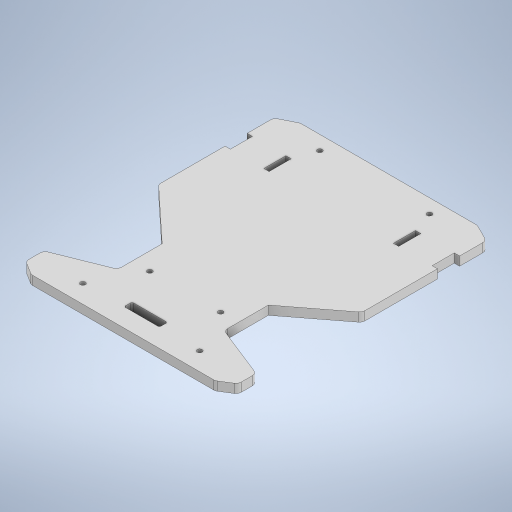
# Autodesk Inventor part: KhungDuoi
Saved by Autodesk Inventor 2023 (Build 270158000, 158)
## iProperties
Created: 2023-03-06
Part Number: KhungDuoi
Material: Generic
Document SubType Name: Modeling
Designer: Admins
Density: 1 g/cm^3
Appearance: Default
Author: Admins
Autodesk Inventor part; units mm, degrees
ref_plane "YZ Plane" through (0, 0, 0) normal (1, 0, 0) x (0, 1, 0)
ref_plane "XZ Plane" through (0, 0, 0) normal (0, 1, 0) x (-1, 0, 0)
ref_plane "XY Plane" through (0, 0, 0) normal (0, 0, 1) x (1, 0, 0)
sketch "Sketch1" plane through (0, 0, 0) normal (0, 1, 0) x (-1, 0, 0)
  line L0 (-60, 75) -> (60, 75)
  line L1 (60, -75) -> (-60, -75)
  line L2 (-60, 75) -> (60, -75) construction
  line L3 (60, 75) -> (-60, -75) construction
  line L4 (-60, -75) -> (-60, -55)
  line L5 (-60, -55) -> (-57, -55)
  line L6 (-60, -55) -> (-57, -55)
  line L7 (-57, -55) -> (-57, -42.5)
  line L8 (-57, -42.5) -> (-60, -42.5)
  line L9 (-60, -42.5) -> (-60, -55)
  line L10 (-57, -42.5) -> (-38.1, -42.5)
  line L11 (-38.1, -42.5) -> (-35.1, -42.5)
  line L12 (-35.1, -42.5) -> (-35.1, -55)
  line L13 (-35.1, -55) -> (-38.1, -55)
  line L14 (-38.1, -55) -> (-38.1, -42.5)
  line L15 (0, 75) -> (0, 64.8)
  line L16 (0, 64.8) -> (-33, 64.8)
  line L17 (-33, 64.8) -> (33, 64.8)
  circle A0 centre (-33, 64.8) radius 1.4
  circle A1 centre (33, 64.8) radius 1.4
  line L18 (0, 75) -> (0, 40)
  line L19 (0, 40) -> (-20, 40)
  line L20 (-20, 40) -> (20, 40)
  circle A2 centre (20, 40) radius 1.4
  circle A3 centre (-20, 40) radius 1.4
  line L21 (-60, -75) -> (-60, -5)
  line L22 (-4, -5) -> (4, -5)
  line L23 (-60, 75) -> (-60, 60)
  line L24 (-60, 60) -> (60, 60)
  line L25 (-20, 40) -> (-21.4, 40)
  line L26 (20, 40) -> (21.4, 40)
  line L27 (-30, 40) -> (-30, 10)
  line L28 (-30, 10) -> (-60, 0)
  line L29 (30, 40) -> (30, 10)
  line L30 (30, 10) -> (60, -5)
  line L31 (-30, 40) -> (-30, 48)
  line L32 (-30, 48) -> (-60, 60)
  line L33 (30, 40) -> (30, 48)
  line L34 (30, 48) -> (60, 60)
  line L35 (0, 75) -> (0, -75)
  line L36 (0, -75) -> (-60, -75)
  line L37 (0, 75) -> (-60, 75)
  line L38 (60, -70) -> (60, -55)
  line L39 (60, -55) -> (57, -55)
  line L40 (57, -55) -> (57, -42.5)
  line L41 (57, -42.5) -> (60, -42.5)
  line L42 (60, -42.5) -> (60, -55)
  line L43 (57, -42.5) -> (38.1, -42.5)
  line L44 (38.1, -42.5) -> (35.1, -42.5)
  line L45 (35.1, -42.5) -> (35.1, -55)
  line L46 (35.1, -55) -> (38.1, -55)
  line L47 (38.1, -55) -> (38.1, -42.5)
  line L48 (60, 75) -> (52, 75)
  line L49 (52, 75) -> (52, 70)
  line L50 (52, 70) -> (60, 70)
  line L51 (60, 70) -> (60, 75)
  line L52 (-60, 75) -> (-52, 75)
  line L53 (-52, 75) -> (-52, 70)
  line L54 (-52, 70) -> (-60, 70)
  line L55 (-60, 70) -> (-60, 75)
  line L56 (60, 70) -> (52, 75)
  line L57 (-52, 75) -> (-60, 70)
  line L58 (60, 75) -> (60, 60)
  line L59 (60, -5) -> (60, -70)
  line L60 (-60, -75) -> (-60, 0)
  line L61 (-60, 60) -> (-60, 75)
  line L62 (57, -75) -> (50, -75)
  line L63 (50, -75) -> (50, -70)
  line L64 (50, -70) -> (60, -70)
  line L65 (60, -70) -> (60, -75)
  line L66 (-60, -75) -> (-50, -75)
  line L67 (-50, -75) -> (-50, -70)
  line L68 (-50, -70) -> (-60, -70)
  line L69 (-60, -70) -> (-60, -75)
  line L70 (-60, -70) -> (-50, -75)
  line L71 (60, -70) -> (50, -75)
  line L72 (33, 64.8) -> (33, 62.8)
  line L73 (33, 62.8) -> (-33, 62.8)
  line L74 (-33, 62.8) -> (-33, 64.8)
  line L75 (0, 62.8) -> (10, 62.8)
  line L76 (10, 62.8) -> (-10, 62.8)
  line L77 (-10, 61.05) -> (10, 61.05)
  line L78 (10, 61.05) -> (10, 64.55)
  line L79 (10, 64.55) -> (-10, 64.55)
  line L80 (-10, 64.55) -> (-10, 61.05)
  line L81 (-10, 61.05) -> (10, 64.55) construction
  line L82 (10, 61.05) -> (-10, 64.55) construction
  line L83 (10, 61.05) -> (-10, 61.05)
  line L84 (-10, 61.05) -> (-10, 60)
  line L85 (-10, 60) -> (10, 60)
  line L86 (10, 60) -> (10, 61.05)
  line L87 (30, 48) -> (30, 23)
  line L88 (30, 23) -> (60, -5)
  line L89 (-30, 48) -> (-30, 23)
  line L90 (-30, 23) -> (-60, 0)
  line L91 (60, -75) -> (31, -75)
  line L92 (31, -75) -> (31, -67)
  line L93 (31, -67) -> (60, -67)
  line L94 (60, -67) -> (60, -75)
  line L95 (-60, -75) -> (-31, -75)
  line L96 (-31, -75) -> (-31, -67)
  line L97 (-31, -67) -> (-60, -67)
  line L98 (-60, -67) -> (-60, -75)
  circle A4 centre (-31, -67) radius 1.4
  circle A5 centre (31, -67) radius 1.4
  point P0 (0, 0)
  dimension "d16" = 2.8
  dimension "d17" = 2.8
  dimension "d0" = 120
  dimension "d1" = 150
  dimension "d2" = 20
  dimension "d3" = 3
  dimension "d4" = 3
  dimension "d5" = 12.5
  dimension "d6" = 18.9
  dimension "d7" = 3
  dimension "d8" = 10.2
  dimension "d9" = 33
  dimension "d10" = 66
  dimension "d11" = 2.8
  dimension "d12" = 2.8
  dimension "d13" = 35
  dimension "d14" = 20
  dimension "d15" = 40
  dimension "d18" = 70
  dimension "d19" = 15
  dimension "d20" = 10
  dimension "d21" = 10
  dimension "d22" = 30
  dimension "d23" = 30
  dimension "d24" = 8
  dimension "d25" = 8
  dimension "d26" = 20
  dimension "d27" = 3
  dimension "d28" = 12.5
  dimension "d29" = 18.9
  dimension "d30" = 3
  dimension "d31" = 8
  dimension "d32" = 5
  dimension "d33" = 8
  dimension "d34" = 5
  dimension "d35" = 10
  dimension "d36" = 5
  dimension "d37" = 10
  dimension "d38" = 5
  dimension "d42" = 2
  dimension "d43" = 10
  dimension "d44" = 20
  dimension "d45" = 3.5
  dimension "d47" = 25
  dimension "d48" = 25
  dimension "d49" = 29
  dimension "d50" = 8
  dimension "d51" = 29
  dimension "d52" = 8
  dimension "d53" = 2.8
  dimension "d54" = 2.8
  constraints: 198 end point, 30 parallel, 23 perpendicular, 17 point on line, 16 horizontal, 7 midpoint, 6 coincident, 4 centre point, 3 vertical, 2 collinear, 2 horizontal alignment, 4 other
  measures "d0" distance of L1.start L1.end
  measures "d1" distance of L0.end L1.start
  measures "d2" distance of L1.end L4.end
  measures "d3" distance of L4.end L5.end
  measures "d4" distance of L8.end L7.end
  measures "d5" distance of L7.end L6.end
  measures "d6" distance of L7.end L10.end
  measures "d7" distance of L12.end L13.end
  measures "d8" distance of L15.start L15.end
  measures "d9" distance of L15.end L16.end
  measures "d10" distance of L16.end L17.end
  measures "d11" diameter of A0
  measures "d12" diameter of A1
  measures "d13" distance of L15.start L18.end
  measures "d14" distance of L18.end L19.end
  measures "d15" distance of L19.end L20.end
  measures "d18" distance of L1.end L21.end
  measures "d19" distance of L0.start L23.end
  measures "d20" distance of L25.start L27.start
  measures "d21" distance of L26.start L29.start
  measures "d22" distance of L27.start L27.end
  measures "d23" distance of L29.start L29.end
  measures "d24" distance of L27.start L31.end
  measures "d25" distance of L29.start L33.end
  measures "d26" distance of L1.start L38.end
  measures "d27" distance of L40.end L41.end
  measures "d28" distance of L39.end L40.end
  measures "d29" distance of L40.end L43.end
  measures "d30" distance of L46.end L45.end
  measures "d31" distance of L50.end L49.end
  measures "d32" distance of L49.end L48.end
  measures "d33" distance of L53.end L54.end
  measures "d34" distance of L52.end L53.end
  measures "d35" distance of L38.start L63.end
  measures "d36" distance of L62.end L63.end
  measures "d37" distance of L68.end L67.end
  measures "d38" distance of L67.end L66.end
  measures "d42" distance of L72.start L72.end
  measures "d43" distance of L75.start L75.end
  measures "d44" distance of L75.end L76.end
  measures "d45" distance of L78.end L77.end
  measures "d47" distance of L33.end L87.end
  measures "d48" distance of L31.end L89.end
  measures "d49" distance of L92.end L93.end
  measures "d50" distance of L91.end L92.end
  measures "d51" distance of L97.end L96.end
  measures "d52" distance of L96.end L95.end
  measures "d53" diameter of A4
  measures "d54" diameter of A5
extrude "Extrusion1" add sketch "Sketch1" along normal blind 5 contours L0 L15 L16 A0 L74 L73 L80 L84 L24 L23 L54 L53 | L53 L54 L57 | L0 L49 L50 L58 L24 L86 L78 L73 L72 A1 L17 L15 | L24 L18 L35 L1 L96 A4 L97 L4 L5 L7 L8 L21 L60 L28 L27 L31 L32 | L56 L50 L49 | L18 L79 L80 L73 L74 A0 L16 | L17 A1 L72 L73 L78 L79 L18 | L24 L34 L33 L29 L30 L59 L41 L40 L39 L38 L93 A5 L92 L1 L35 L18 | L27 L28 L90 | L88 L30 L29 | L92 A5 L93 L38 L64 L63 L1 | L1 L67 L68 L4 L97 A4 L96 | L63 L64 L71 | L70 L68 L67
fillet "Fillet1" radius 3 14 edges at (-52, 2.5, 75) (-60, 2.5, 70) (-60, 2.5, 60) (-30, 2.5, 48) (-60, 2.5, -5) (-50, 2.5, -75) (-60, 2.5, -70) (60, 2.5, -70) (50, 2.5, -75) (60, 2.5, 0) (30, 2.5, 48) (52, 2.5, 75) (60, 2.5, 70) (60, 2.5, 60)
fillet "Fillet2" radius 1 4 edges at (-10, 2.5, 64.55) (-10, 2.5, 60) (10, 2.5, 64.55) (10, 2.5, 60)
body "Solid1"
